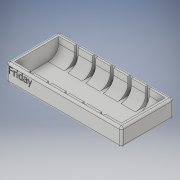
# Autodesk Inventor part: Friday
Saved by Autodesk Inventor 2019.4 (Build 234330000, 330)
## iProperties
Created: 2020-10-20
Part Number: Friday
Material: Generic
Document SubType Name: Modeling
Designer: daanswinters
Density: 1 g/cm^3
Appearance: Default
Author: daanswinters
Autodesk Inventor part; units mm, degrees
ref_plane "YZ Plane" through (0, 0, 0) normal (1, 0, 0) x (0, 1, 0)
ref_plane "XZ Plane" through (0, 0, 0) normal (0, 1, 0) x (-1, 0, 0)
ref_plane "XY Plane" through (0, 0, 0) normal (0, 0, 1) x (1, 0, 0)
sketch "Sketch1" plane through (0, 0, 0) normal (0, 0, 1) x (1, 0, 0)
  line L0 (55, -8.5) -> (-55, -8.5)
  line L1 (-55, -8.5) -> (-55, 8.5)
  line L2 (-55, 8.5) -> (55, 8.5)
  line L3 (55, 8.5) -> (55, -8.5)
  line L4 (55, -8.5) -> (-55, 8.5) construction
  line L5 (-55, -8.5) -> (55, 8.5) construction
  point P0 (0, 0)
  dimension "d0" = 110
  dimension "d1" = 17
  constraints: 12 end point, 2 midpoint, 2 parallel, 1 horizontal, 1 perpendicular
  measures "d0" distance of L1.end L2.end
  measures "d1" distance of L0.end L1.end
extrude "Extrusion1" add sketch "Sketch1" along normal blind 50
sketch "Sketch2" plane through (-55, 8.5, 0) normal (0, 1, 0) x (1, 0, 0)
  line L0 (0, 0) -> (0, -50) projected
  line L1 (110, -50) -> (0, -50)
  line L2 (0, -50) -> (0, 0)
  line L3 (0, 0) -> (110, 0)
  line L4 (110, 0) -> (110, -50)
  line L5 (110, -50) -> (0, 0) construction
  line L6 (0, -50) -> (110, 0) construction
  line L7 (106, -46) -> (106, -4)
  line L8 (4, -4) -> (4, -46)
  line L9 (56.15, -2) -> (53.85, -2)
  line L10 (53.85, -48) -> (56.15, -48)
  line L11 (56.15, -2) -> (53.85, -48) construction
  line L12 (53.85, -2) -> (56.15, -48) construction
  line L13 (73.15, -2) -> (70.85, -2)
  line L14 (70.85, -48) -> (73.15, -48)
  line L15 (73.15, -2) -> (70.85, -48) construction
  line L16 (70.85, -2) -> (73.15, -48) construction
  line L17 (0, -25) -> (110, -25) construction
  line L18 (87.85, -2) -> (90.15, -2)
  line L19 (90.15, -48) -> (87.85, -48)
  line L20 (87.85, -2) -> (90.15, -48) construction
  line L21 (90.15, -2) -> (87.85, -48) construction
  line L22 (36.85, -2) -> (39.15, -2)
  line L23 (39.15, -48) -> (36.85, -48)
  line L24 (36.85, -2) -> (39.15, -48) construction
  line L25 (39.15, -2) -> (36.85, -48) construction
  line L26 (19.85, -2) -> (22.15, -2)
  line L27 (22.15, -48) -> (19.85, -48)
  line L28 (19.85, -2) -> (22.15, -48) construction
  line L29 (22.15, -2) -> (19.85, -48) construction
  line L30 (90.15, -2) -> (90.15, -4)
  line L31 (90.15, -46) -> (90.15, -48)
  line L32 (87.85, -48) -> (87.85, -46)
  line L33 (87.85, -4) -> (87.85, -2)
  line L34 (73.15, -48) -> (73.15, -46)
  line L35 (73.15, -4) -> (73.15, -2)
  line L36 (70.85, -2) -> (70.85, -4)
  line L37 (70.85, -46) -> (70.85, -48)
  line L38 (56.15, -4) -> (56.15, -2)
  line L39 (53.85, -2) -> (53.85, -4)
  line L40 (53.85, -46) -> (53.85, -48)
  line L41 (56.15, -48) -> (56.15, -46)
  line L42 (39.15, -2) -> (39.15, -4)
  line L43 (39.15, -46) -> (39.15, -48)
  line L44 (36.85, -48) -> (36.85, -46)
  line L45 (36.85, -4) -> (36.85, -2)
  line L46 (22.15, -2) -> (22.15, -4)
  line L47 (19.85, -48) -> (19.85, -46)
  line L48 (19.85, -4) -> (19.85, -2)
  line L49 (22.15, -46) -> (22.15, -48)
  line L50 (4, -46) -> (19.95, -46)
  line L51 (22.05, -46) -> (36.95, -46)
  line L52 (39.05, -46) -> (53.95, -46)
  line L53 (56.05, -46) -> (70.95, -46)
  line L54 (73.05, -46) -> (87.95, -46)
  line L55 (90.05, -46) -> (106, -46)
  line L56 (106, -4) -> (90.05, -4)
  line L57 (87.95, -4) -> (73.05, -4)
  line L58 (70.95, -4) -> (56.05, -4)
  line L59 (53.95, -4) -> (39.05, -4)
  line L60 (36.95, -4) -> (22.05, -4)
  line L61 (19.95, -4) -> (4, -4)
  point P0 (55, 0)
  point P1 (55, -25)
  point P2 (72, -25)
  point P3 (89, -25)
  point P4 (38, -25)
  point P5 (21, -25)
  dimension "d4" = 65.556
  dimension "d5" = 110
  dimension "d7" = 2.3
  dimension "d8" = 46
  dimension "d9" = 2.3
  dimension "d10" = 46
  dimension "d11" = 0
  dimension "d12" = 2.3
  dimension "d13" = 46
  dimension "d14" = 2.3
  dimension "d15" = 46
  dimension "d16" = 2.3
  dimension "d17" = 46
  dimension "d18" = 17
  dimension "d19" = 17
  dimension "d20" = 17
  dimension "d21" = 17
  dimension "d22" = 2.862
  dimension "d23" = 2.862
  dimension "d24" = 106
  dimension "d25" = 4
  dimension "d26" = 42
  dimension "d27" = 2
  dimension "d28" = 0
  dimension "d29" = 42
  dimension "d30" = 0
  dimension "d31" = 42
  dimension "d32" = 0
  dimension "d33" = 42
  dimension "d34" = 0
  dimension "d35" = 42
  dimension "d36" = 0
  dimension "d37" = 42
  constraints: 122 end point, 73 parallel, 43 point on line, 17 perpendicular, 14 midpoint, 6 horizontal
  measures "d4" angle of L5 L0
  measures "d5" distance between parallel lines of L4 L0
  measures "d7" distance of L10.end L10.start
  measures "d8" distance of L10.start L9.end
  measures "d9" distance of L14.end L14.start
  measures "d10" distance of L14.start L13.end
  measures "d11" distance from line of L17 point (72, -25)
  measures "d12" distance of L19.start L19.end
  measures "d13" distance of L18.end L19.start
  measures "d14" distance of L23.start L23.end
  measures "d15" distance of L22.end L23.start
  measures "d16" distance of L27.start L27.end
  measures "d17" distance of L26.end L27.start
  measures "d18" distance of point (72, -25) point (55, -25)
  measures "d19" distance of point (89, -25) point (72, -25)
  measures "d20" distance of point (38, -25) point (55, -25)
  measures "d21" distance of point (21, -25) point (38, -25)
  measures "d22" angle of L0 L20
  measures "d23" angle of L0 L21
  measures "d24" distance between parallel lines of L7 L0
  measures "d25" distance between parallel lines of L8 L0
  measures "d26" distance between parallel lines of L56 L55
  measures "d27" distance between parallel lines of L56 L18
  measures "d28" distance between parallel lines of L56 L57
  measures "d29" distance between parallel lines of L56 L54
  measures "d30" distance between parallel lines of L56 L58
  measures "d31" distance between parallel lines of L56 L53
  measures "d32" distance between parallel lines of L56 L59
  measures "d33" distance between parallel lines of L56 L52
  measures "d34" distance between parallel lines of L56 L60
  measures "d35" distance between parallel lines of L56 L51
  measures "d36" distance between parallel lines of L56 L61
  measures "d37" distance between parallel lines of L56 L50
extrude "Extrusion2" cut sketch "Sketch2" against normal blind 16 contours L55 L31 L19 L32 L54 L34 L14 L37 L53 L41 L10 L40 L52 L43 L23 L44 L51 L49 L27 L47 L50 L8 L61 L48 L26 L46 L60 L45 L22 L42 L59 L39 L9 L38 L58 L36 L13 L35 L57 L33 L18 L30 L56 L7
fillet "Fillet1" radius 2 12 edges at (-55, 0, 50) (-55, 0, 0) (55, 0, 50) (55, 0, 0) (0, 8.5, 50) (-55, 8.5, 25) (0, 8.5, 0) (55, 8.5, 25) (55, -8.5, 25) (0, -8.5, 50) (-55, -8.5, 25) (0, -8.5, 0)
fillet "Fillet2" radius 10 6 edges at (-43.075, -7.5, 4) (-25.5, -7.5, 4) (-8.5, -7.5, 4) (8.5, -7.5, 4) (25.5, -7.5, 4) (43.075, -7.5, 4)
sketch "Sketch3" plane through (35.15, 8.5, 4) normal (0, 1, 0) x (1, 0, 0)
  line L0 (-70.3, -44) -> (-70.3, -42) projected
  line L1 (-51, 2) -> (-53.3, 2)
  line L2 (-34, 2) -> (-34, 0) projected
  line L3 (-36.3, -44) -> (-36.3, -42) projected
  line L4 (-19.3, -44) -> (-19.3, -42) projected
  line L5 (-2.3, -44) -> (-2.3, -42) projected
  line L6 (0, 2) -> (0, 0) projected
  line L7 (-19.8, 2) -> (-16.5, 2)
  line L8 (-16.5, 2) -> (-16.5, -44)
  line L9 (-16.5, -44) -> (-19.8, -44)
  line L10 (-19.8, -44) -> (-19.8, 2)
  line L11 (-19.8, 2) -> (-16.5, -44) construction
  line L12 (-16.5, 2) -> (-19.8, -44) construction
  line L13 (-2.8, -44) -> (0.5, -44)
  line L14 (0.5, -44) -> (0.5, 2)
  line L15 (0.5, 2) -> (-2.8, 2)
  line L16 (-2.8, 2) -> (-2.8, -44)
  line L17 (-2.8, -44) -> (0.5, 2) construction
  line L18 (0.5, -44) -> (-2.8, 2) construction
  line L19 (-36.8, -44) -> (-33.5, -44)
  line L20 (-33.5, -44) -> (-33.5, 2)
  line L21 (-33.5, 2) -> (-36.8, 2)
  line L22 (-36.8, 2) -> (-36.8, -44)
  line L23 (-36.8, -44) -> (-33.5, 2) construction
  line L24 (-33.5, -44) -> (-36.8, 2) construction
  line L25 (-51, 2) -> (-36.3, 2) projected
  line L26 (-53.8, -44) -> (-50.5, -44)
  line L27 (-50.5, -44) -> (-50.5, 2)
  line L28 (-50.5, 2) -> (-53.8, 2)
  line L29 (-53.8, 2) -> (-53.8, -44)
  line L30 (-53.8, -44) -> (-50.5, 2) construction
  line L31 (-50.5, -44) -> (-53.8, 2) construction
  line L32 (-53.3, -44) -> (-68, -44) projected
  line L33 (-70.8, 2) -> (-67.5, 2)
  line L34 (-67.5, 2) -> (-67.5, -44)
  line L35 (-67.5, -44) -> (-70.8, -44)
  line L36 (-70.8, -44) -> (-70.8, 2)
  line L37 (-70.8, 2) -> (-67.5, -44) construction
  line L38 (-67.5, 2) -> (-70.8, -44) construction
  point P0 (-35.15, 4)
  point P1 (-68, 2)
  point P2 (-17, 2)
  point P3 (-18.15, -21)
  point P4 (-1.15, -21)
  point P5 (-35.15, -21)
  point P6 (-52.15, -21)
  point P7 (-69.15, -21)
  dimension "d42" = 3.3
  dimension "d43" = 46
  dimension "d44" = 3.3
  dimension "d45" = 3.3
  dimension "d46" = 3.3
  dimension "d47" = 3.3
  dimension "d48" = 90
  dimension "d49" = 0.5
  dimension "d50" = 16.5
  dimension "d51" = 33.5
  dimension "d52" = 50.5
  dimension "d53" = 67.5
  dimension "d54" = 46
  dimension "d55" = 0
  dimension "d56" = 53.3
  constraints: 62 end point, 14 parallel, 10 midpoint, 5 horizontal, 5 perpendicular, 3 point on line
  measures "d42" distance of L8.end L9.end
  measures "d43" distance of L7.end L8.end
  measures "d44" distance of L15.end L14.end
  measures "d45" distance of L21.end L20.end
  measures "d46" distance of L28.end L27.end
  measures "d47" distance of L34.end L35.end
  measures "d48" angle of L6 L1
  measures "d49" distance between parallel lines of L6 L14
  measures "d50" distance between parallel lines of L6 L8
  measures "d51" distance between parallel lines of L6 L20
  measures "d52" distance between parallel lines of L6 L27
  measures "d53" distance between parallel lines of L6 L34
  measures "d54" distance between parallel lines of L25 L9
  measures "d55" distance between parallel lines of L15 L25
  measures "d56" distance from line of L1.end L6
extrude "Extrusion3" cut sketch "Sketch3" against normal blind 16
sketch "Sketch4" plane through (0, 0, 50) normal (0, 0, 1) x (1, 0, 0)
  line L0 (-52.9749, 6.5012) -> (53.0345, 6.5012) construction
  line L1 (53.0345, 6.5012) -> (53.0345, -6.5247) construction
  line L2 (53.0345, -6.5247) -> (-52.9749, -6.5247) construction
  line L3 (-52.9749, -6.5247) -> (-52.9749, 6.5012) construction
  line L4 (-48.7089, 5.5077) -> (-51.5463, 5.5077)
  line L5 (-51.5463, 5.5077) -> (-51.5463, 3.7874)
  line L6 (-51.5463, 3.7874) -> (-48.8275, 3.7874)
  line L7 (-48.8275, 3.7874) -> (-48.8275, 3.0657)
  line L8 (-48.8275, 3.0657) -> (-51.5463, 3.0657)
  line L9 (-51.5463, 3.0657) -> (-51.5463, 0.1294)
  line L10 (-51.5463, 0.1294) -> (-52.357, 0.1294)
  line L11 (-52.357, 0.1294) -> (-52.357, 6.2294)
  line L12 (-52.357, 6.2294) -> (-48.7089, 6.2294)
  line L13 (-48.7089, 6.2294) -> (-48.7089, 5.5077)
  line L14 (-45.6144, 3.8813) -> (-45.6539, 3.8813)
  spline S0 degree 2 poles (-45.6539, 3.8813) (-45.7429, 3.906) (-45.9357, 3.9159) (-46.0692, 3.9159) knots 0 0 0 1 2 2 2
  spline S1 degree 2 poles (-46.0692, 3.9159) (-46.3806, 3.9159) (-46.9936, 3.644) (-47.2704, 3.3771) knots 0 0 0 1 2 2 2
  line L15 (-47.2704, 3.3771) -> (-47.2704, 0.1294)
  line L16 (-47.2704, 0.1294) -> (-48.0415, 0.1294)
  line L17 (-48.0415, 0.1294) -> (-48.0415, 4.7068)
  line L18 (-48.0415, 4.7068) -> (-47.2704, 4.7068)
  line L19 (-47.2704, 4.7068) -> (-47.2704, 4.0247)
  spline S2 degree 2 poles (-47.2704, 4.0247) (-46.8502, 4.4004) (-46.2224, 4.7068) (-45.9258, 4.7068) knots 0 0 0 1 2 2 2
  spline S3 degree 2 poles (-45.9258, 4.7068) (-45.8072, 4.7068) (-45.6885, 4.697) (-45.6144, 4.6821) knots 0 0 0 1 2 2 2
  line L20 (-45.6144, 4.6821) -> (-45.6144, 3.8813)
  line L21 (-44.2303, 0.1294) -> (-45.0014, 0.1294)
  line L22 (-45.0014, 0.1294) -> (-45.0014, 4.7068)
  line L23 (-45.0014, 4.7068) -> (-44.2303, 4.7068)
  line L24 (-44.2303, 4.7068) -> (-44.2303, 0.1294)
  line L25 (-44.1759, 5.4681) -> (-45.0509, 5.4681)
  line L26 (-45.0509, 5.4681) -> (-45.0509, 6.2689)
  line L27 (-45.0509, 6.2689) -> (-44.1759, 6.2689)
  line L28 (-44.1759, 6.2689) -> (-44.1759, 5.4681)
  line L29 (-39.5787, 0.1294) -> (-40.3498, 0.1294)
  line L30 (-40.3498, 0.1294) -> (-40.3498, 0.594)
  spline S4 degree 2 poles (-40.3498, 0.594) (-40.5278, 0.4457) (-40.7898, 0.248) (-40.9677, 0.164) knots 0 0 0 1 2 2 2
  spline S5 degree 2 poles (-40.9677, 0.164) (-41.1308, 0.0849) (-41.4818, 0.0008) (-41.7141, 0.0008) knots 0 0 0 1 2 2 2
  spline S6 degree 2 poles (-41.7141, 0.0008) (-42.0898, 0.0008) (-42.7226, 0.3123) (-42.945, 0.6138) knots 0 0 0 1 2 2 2
  spline S7 degree 2 poles (-42.945, 0.6138) (-43.1675, 0.9153) (-43.4146, 1.8051) (-43.4146, 2.3835) knots 0 0 0 1 2 2 2
  spline S8 degree 2 poles (-43.4146, 2.3835) (-43.4146, 2.9866) (-43.1032, 3.8665) (-42.8313, 4.1977) knots 0 0 0 1 2 2 2
  spline S9 degree 2 poles (-42.8313, 4.1977) (-42.5792, 4.4943) (-41.8723, 4.8354) (-41.4818, 4.8354) knots 0 0 0 1 2 2 2
  spline S10 degree 2 poles (-41.4818, 4.8354) (-41.1407, 4.8354) (-40.6316, 4.6821) (-40.3498, 4.5239) knots 0 0 0 1 2 2 2
  line L31 (-40.3498, 4.5239) -> (-40.3498, 6.5012)
  line L32 (-40.3498, 6.5012) -> (-39.5787, 6.5012)
  line L33 (-39.5787, 6.5012) -> (-39.5787, 0.1294)
  line L34 (-40.3498, 1.2416) -> (-40.3498, 3.8863)
  spline S11 degree 2 poles (-40.3498, 3.8863) (-40.6365, 4.0247) (-41.0913, 4.1285) (-41.3533, 4.1285) knots 0 0 0 1 2 2 2
  spline S12 degree 2 poles (-41.3533, 4.1285) (-41.9465, 4.1285) (-42.6188, 3.2387) (-42.6188, 2.3983) knots 0 0 0 1 2 2 2
  spline S13 degree 2 poles (-42.6188, 2.3983) (-42.6188, 1.5876) (-42.1047, 0.7324) (-41.5362, 0.7324) knots 0 0 0 1 2 2 2
  spline S14 degree 2 poles (-41.5362, 0.7324) (-41.2347, 0.7324) (-40.6217, 1.0093) (-40.3498, 1.2416) knots 0 0 0 1 2 2 2
  spline S15 degree 2 poles (-35.9107, 0.6138) (-36.0047, 0.5446) (-36.321, 0.2974) (-36.4693, 0.2233) knots 0 0 0 1 2 2 2
  spline S16 degree 2 poles (-36.4693, 0.2233) (-36.672, 0.1145) (-37.0526, 0.0008) (-37.3987, 0.0008) knots 0 0 0 1 2 2 2
  spline S17 degree 2 poles (-37.3987, 0.0008) (-37.6804, 0.0008) (-38.1896, 0.2134) (-38.3824, 0.4062) knots 0 0 0 1 2 2 2
  spline S18 degree 2 poles (-38.3824, 0.4062) (-38.5653, 0.594) (-38.7877, 1.1477) (-38.7877, 1.4542) knots 0 0 0 1 2 2 2
  spline S19 degree 2 poles (-38.7877, 1.4542) (-38.7877, 1.9287) (-38.3873, 2.601) (-37.9523, 2.7938) knots 0 0 0 1 2 2 2
  spline S20 degree 2 poles (-37.9523, 2.7938) (-37.5667, 2.9718) (-36.5188, 3.1052) (-35.9107, 3.1398) knots 0 0 0 1 2 2 2
  line L35 (-35.9107, 3.1398) -> (-35.9107, 3.2881)
  spline S21 degree 2 poles (-35.9107, 3.2881) (-35.9107, 3.5551) (-36.0739, 3.8863) (-36.2222, 3.9802) knots 0 0 0 1 2 2 2
  spline S22 degree 2 poles (-36.2222, 3.9802) (-36.3705, 4.0741) (-36.7956, 4.1334) (-37.023, 4.1334) knots 0 0 0 1 2 2 2
  spline S23 degree 2 poles (-37.023, 4.1334) (-37.2899, 4.1334) (-38.0116, 3.9752) (-38.3725, 3.822) knots 0 0 0 1 2 2 2
  line L36 (-38.3725, 3.822) -> (-38.417, 3.822)
  line L37 (-38.417, 3.822) -> (-38.417, 4.608)
  spline S24 degree 2 poles (-38.417, 4.608) (-38.2044, 4.6673) (-37.4086, 4.8156) (-37.018, 4.8156) knots 0 0 0 1 2 2 2
  spline S25 degree 2 poles (-37.018, 4.8156) (-36.5435, 4.8156) (-35.8959, 4.6673) (-35.6389, 4.4745) knots 0 0 0 1 2 2 2
  spline S26 degree 2 poles (-35.6389, 4.4745) (-35.3868, 4.2867) (-35.1396, 3.6885) (-35.1396, 3.2585) knots 0 0 0 1 2 2 2
  line L38 (-35.1396, 3.2585) -> (-35.1396, 0.1294)
  line L39 (-35.1396, 0.1294) -> (-35.9107, 0.1294)
  line L40 (-35.9107, 0.1294) -> (-35.9107, 0.6138)
  line L41 (-35.9107, 1.2564) -> (-35.9107, 2.5269)
  spline S27 degree 2 poles (-35.9107, 2.5269) (-36.1876, 2.5021) (-37.023, 2.4181) (-37.285, 2.339) knots 0 0 0 1 2 2 2
  spline S28 degree 2 poles (-37.285, 2.339) (-37.5915, 2.2451) (-37.9919, 1.8546) (-37.9919, 1.5085) knots 0 0 0 1 2 2 2
  spline S29 degree 2 poles (-37.9919, 1.5085) (-37.9919, 1.1131) (-37.547, 0.7127) (-37.1218, 0.7127) knots 0 0 0 1 2 2 2
  spline S30 degree 2 poles (-37.1218, 0.7127) (-36.761, 0.7127) (-36.1678, 1.0241) (-35.9107, 1.2564) knots 0 0 0 1 2 2 2
  line L42 (-30.4633, 4.7068) -> (-32.925, -1.5563)
  line L43 (-32.925, -1.5563) -> (-33.7505, -1.5563)
  line L44 (-33.7505, -1.5563) -> (-32.93, 0.3518)
  line L45 (-32.93, 0.3518) -> (-34.5909, 4.7068)
  line L46 (-34.5909, 4.7068) -> (-33.7604, 4.7068)
  line L47 (-33.7604, 4.7068) -> (-32.5098, 1.3158)
  line L48 (-32.5098, 1.3158) -> (-31.2641, 4.7068)
  line L49 (-31.2641, 4.7068) -> (-30.4633, 4.7068)
  point P0 (0, 0)
  constraints: 2 other
extrude "Extrusion4" cut sketch "Sketch4" against normal blind 0.5
fillet "Fillet3" radius 10 6 edges at (-43.325, -7.5, 46) (-25.5, -7.5, 46) (-8.5, -7.5, 46) (8.5, -7.5, 46) (25.5, -7.5, 46) (43.325, -7.5, 46)
body "Solid1"
